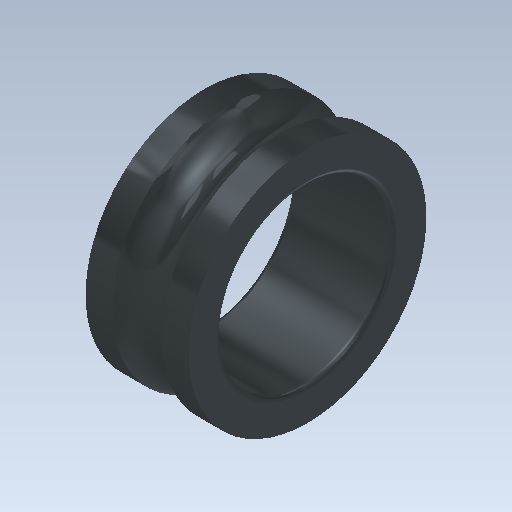
# Autodesk Inventor part: 6900ZZ Inner Ring
Saved by Autodesk Inventor 2021 (Build 250183000, 183)
## iProperties
Category: PARTsolutions
Company: NTN
Created: 2019-07-31
Part Number: 6900ZZ Inner Ring
Material: 鉄、鋳鉄
Catalog Web Link: www.cadenas.de
Description: Open type ir-Deep Groove Ball Bearings
Vendor: NTN
Document SubType Name: Modeling
Designer: psadmin
Manufacturer: NTN
Mass: 2.64428 g
Surface Area: 5.95169 cm^2
Volume: 0.36983 cm^3
Density: 7.15 g/cm^3
Appearance: 鉄 灰色
PSOL_IDENT_0: {$CADENAS_DATA\23d-libs\ntn\ball_roller_bearings\deep_groove_bb\deep_groove_bb\6_types\dgbb_ir.prj},
PSOL_IDENT_1: 182 {VTYP=3D},{NB=6900ZZ Inner Ring},{LINA=6900ZZ Inner Ring},{NN=Open type ir},{DATE=29.01.2019 23:
PSOL_IDENT_2: 03:43},{GEOMDATE=14.01.2008 00:00:00},{VERSION=},{LINEID=2800},{WBVAR=},{WBNUMERIC=}  {NB=6900ZZ Inn
PSOL_IDENT_3: er Ring},{LINA=6900ZZ Inner Ring},{KT=DUMMY},{IDNR=},{SD=10},{D=22},{B=6},{R=0.3},{ORDER1=6900},{ORD
PSOL_IDENT_4: ER=6900ZZ},{CR=2.70},{COR=1.27},{CRF=275},{CORF=129},{LSG=30000},{LSO=36000},{MASS=0.01},{RNS=0.3},{
PSOL_IDENT_5: LLH=0},{LLU=21000},{ST=ZZ},{NCST=LLB},{LTST=0},{CST=LLU},{SRG=N},{SR=NR},{D1=20.80},{A=1.05},{BA=0.8
PSOL_IDENT_6: 0},{R0=0.20},{D2=24.8},{F=0.70},{DA1=12},{DA2=13},{DA=20},{DX=25.5},{CY=1.5},{CZ=0.7},{RAS=0.3},{RNA
PSOL_IDENT_7: S=0.3},{VERS=2},{X=6}
NN: Open type ir
NT: Deep Groove Ball Bearings
NB: 6900ZZ Inner Ring
NBSYN: $ORDER. Inner Ring
LINA: 6900ZZ Inner Ring
SD: 10
D: 22
B: 6
R: 0.3
ORDER1: 6900
CR: 2.70
COR: 1.27
CRF: 275
CORF: 129
LSG: 30000
LSO: 36000
MASS: 0.01
RNS: 0.3
LLH: 0
LLU: 21000
ST: ZZ
NCST: LLB
LTST: 0
CST: LLU
SRG: N
SR: NR
D1: 0
A: 1.05
BA: 0.8
R0: 0.2
D2: 24.8
F: 0.7
DA1: 12
DA2: 13
DA: 20
DX: 25.5
CY: 1.5
CZ: 0.7
RAS: 0.3
RNAS: 0.3
VERS: 2
SUPPLIER: NTN
ARTICLENO: 6900ZZ Inner Ring
BOMINFO: 6900ZZ Inner Ring
CREATOR: CADENAS GmbH
Title: 6900ZZ Inner Ring
Author: Cadenas PARTsolutions
Comments: Deep Groove Ball Bearings
Autodesk Inventor part; units mm, degrees
sketch "Sketch_1" plane through (0, 0, 0) normal (0, 0, 1) x (1, 0, 0)
  line L0 (6, 0) -> (0, 0)
  arc A0 (0, 5.3) -> (0.3, 5) centre (0.3, 5.3) ccw
  line L1 (0.3, 5) -> (5.7, 5)
  arc A1 (5.7, 5) -> (6, 5.3) centre (5.7, 5.3) ccw
  line L2 (6, 5.3) -> (6, 6.92)
  line L3 (6, 6.92) -> (4.44, 6.92)
  arc A2 (1.56, 6.92) -> (4.44, 6.92) centre (3, 8) ccw
  line L4 (1.56, 6.92) -> (0, 6.92)
  line L5 (0, 6.92) -> (0, 5.3)
  constraints: 12 end point, 6 point on circle, 3 centre point
revolve "Revolution1" add sketch "Sketch_1" angle 360 about axis through (6, 0, 0) along (1, 0, 0)
ref_plane "dgbb_ir_XY" through (0, 0, 0) normal (1, 0, 0) x (0, 0, -1)
ref_plane "dgbb_ir_YZ" through (0, 0, 0) normal (0, 0, -1) x (0, 1, 0)
ref_plane "dgbb_ir_ZX" through (0, 0, 0) normal (0, 1, 0) x (1, 0, 0)
body "Solid1"
